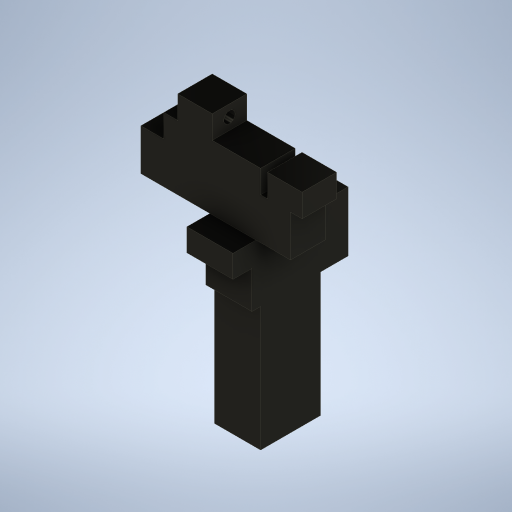
# Autodesk Inventor part: micromanipulator
Saved by Autodesk Inventor 2024 (Build 280153000, 153)
## iProperties
Created: 2021-02-04
Part Number: micromanipulator
Material: Generic
Document SubType Name: Modeling
Designer: Daniel
Density: 1 g/cm^3
Appearance: Gunmetal
Author: Daniel
Autodesk Inventor part; units mm, degrees
ref_plane "YZ Plane" through (0, 0, 0) normal (1, 0, 0) x (0, 1, 0)
ref_plane "XZ Plane" through (0, 0, 0) normal (0, 1, 0) x (-1, 0, 0)
ref_plane "XY Plane" through (0, 0, 0) normal (0, 0, 1) x (1, 0, 0)
sketch "Sketch4" plane through (0, 0, 0) normal (0, 0, 1) x (1, 0, 0)
  line L0 (0, 0) -> (20, 0)
  line L1 (20, 0) -> (20, 54)
  line L2 (20, 54) -> (0, 54)
  line L3 (0, 54) -> (0, 0)
  dimension "d18" = 20
  dimension "d19" = 54
  constraints: 8 end point, 2 parallel, 1 horizontal, 1 perpendicular
  measures "d18" distance of L2.end L1.end
  measures "d19" distance of L1.end L0.end
extrude "Extrusion4" add sketch "Sketch4" along normal mid plane 26
sketch "Sketch5" plane through (0, 54, 13) normal (0, 1, 0) x (1, 0, 0)
  line L0 (0, -12) -> (20, -12)
  line L1 (20, -12) -> (20, 38)
  line L2 (20, 38) -> (0, 38)
  line L3 (0, 38) -> (0, -12)
  line L4 (20, 26) -> (20, 0) projected
  line L5 (0, 26) -> (0, 0) projected
  point P0 (0, 13)
  point P1 (10, 38)
  point P2 (0, 13)
  dimension "d22" = 20
  dimension "d23" = 50
  dimension "d24" = 25
  constraints: 8 end point, 2 midpoint, 2 parallel, 1 collinear, 1 horizontal, 1 perpendicular
  measures "d22" distance between parallel lines of L1 L3
  measures "d23" distance from line of point (10, 38) L0
  measures "d24" distance from line of L0 point (0, 13)
extrude "Extrusion5" add sketch "Sketch5" along normal blind 26
sketch "Sketch6" plane through (0, 0, 0) normal (0, 0, 1) x (1, 0, 0)
  line L0 (35, 80) -> (-30, 80)
  line L1 (-30, 80) -> (-30, 98)
  line L2 (-30, 98) -> (35, 98)
  line L3 (35, 98) -> (35, 80)
  line L4 (0, 80) -> (20, 80) projected
  line L5 (20, 54) -> (20, 80) projected
  line L6 (0, 54) -> (0, 80) projected
  line L7 (-20, 98) -> (22, 98)
  line L8 (22, 98) -> (22, 108)
  line L9 (22, 108) -> (-20, 108)
  line L10 (-20, 108) -> (-20, 98)
  line L11 (25, 98) -> (40, 98)
  line L12 (40, 98) -> (40, 108)
  line L13 (40, 108) -> (25, 108)
  line L14 (25, 108) -> (25, 98)
  line L15 (-14, 108) -> (1, 108)
  line L16 (1, 108) -> (1, 118)
  line L17 (1, 118) -> (-14, 118)
  line L18 (-14, 118) -> (-14, 108)
  point P0 (0, 0)
  point P1 (35, 98)
  point P2 (22, 98)
  point P3 (-20, 103)
  point P4 (-14, 113)
  dimension "d27" = 18
  dimension "d28" = 15
  dimension "d29" = 30
  dimension "d32" = 10
  dimension "d33" = 10
  dimension "d34" = 15
  dimension "d38" = 3
  dimension "d39" = 15
  dimension "d40" = 5
  dimension "d41" = 10
  dimension "d42" = 6
  constraints: 32 end point, 8 parallel, 4 horizontal, 4 perpendicular, 4 point on line, 2 midpoint, 1 collinear
  measures "d27" distance of L0.end L1.end
  measures "d28" distance between parallel lines of L5 L3
  measures "d29" distance between parallel lines of L6 L1
  measures "d32" distance of L9.end L7.start
  measures "d33" distance of L17.end L15.start
  measures "d34" distance of L16.end L17.end
  measures "d38" distance between parallel lines of L8 L14
  measures "d39" distance of L12.end L13.end
  measures "d40" distance between parallel lines of L3 L12
  measures "d41" distance between parallel lines of L1 L10
  measures "d42" horizontal distance of point (-20, 103) point (-14, 113)
extrude "Extrusion6" add sketch "Sketch6" along normal blind 15
sketch "Sketch9" plane through (0, 0, 13) normal (0, 0, 1) x (1, 0, 0)
  point P0 (0, 0)
  point P1 (10, 29.6336)
sketch "Sketch10" plane through (0, 0, 15) normal (0, 0, 1) x (1, 0, 0)
  point P0 (0, 0)
  point P1 (-8.9634, 87.1554)
sketch "Sketch11" plane through (40, 98, 15) normal (1, 0, 0) x (0, 0, -1)
  point P0 (15, -98)
  point P1 (7.5, 5)
sketch "Sketch12" plane through (20, 0, 13) normal (1, 0, 0) x (0, 0, -1)
  point P0 (13, 0)
  point P1 (13, 63.2643)
sketch "Sketch13" plane through (-14, 108, 15) normal (-1, 0, 0) x (0, 0, 1)
  circle A0 centre (-7.5, 5) radius 2.5
  line L0 (-15, 10) -> (0, 10) projected
  line L1 (0, -10) -> (0, 0) projected
  line L2 (-15, 10) -> (0, 0) construction
  point P0 (-15, -108)
  dimension "d35" = 5
  constraints: 2 end point, 1 centre point, 1 midpoint
  measures "d35" diameter of A0
extrude "Extrusion7" cut sketch "Sketch13" against normal through all
sketch "Sketch14" plane through (20, 0, 13) normal (1, 0, 0) x (0, 0, -1)
  line L0 (-31.824, 26.3525) -> (-3.7474, 26.3525)
  line L1 (-3.7474, 26.3525) -> (-3.7474, 70.1914)
  line L2 (-3.7474, 70.1914) -> (-31.824, 70.1914)
  line L3 (-31.824, 70.1914) -> (-31.824, 26.3525)
  line L4 (-31.824, 26.3525) -> (-3.7474, 70.1914) construction
  line L5 (-3.7474, 26.3525) -> (-31.824, 70.1914) construction
  point P0 (13, 0)
  point P1 (-17.7857, 48.272)
  constraints: 12 end point, 2 midpoint, 2 parallel, 1 horizontal, 1 perpendicular
extrude "Extrusion8" cut sketch "Sketch14" against normal through all
equation "\"d24\" = 0.5 * d23"
body "Solid2"
